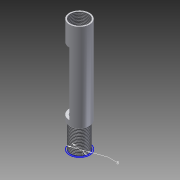
# Autodesk Inventor part: PEEKAufsatz1
Saved by Autodesk Inventor 2012 (Build 160160000, 160)
## iProperties
Created: 2014-06-23
Part Number: PEEKAufsatz1
Material: Polyaryletherketon-Kunststoff
Document SubType Name: Modeling
Designer: kathrin.ganzhorn
Density: 1.32 g/cm^3
Mass: 0.946631 g
Surface Area: 20.3493 cm^2
Volume: 0.717145 cm^3
Author: kathrin.ganzhorn
Autodesk Inventor part; units mm, degrees
ref_plane "YZ Plane" through (0, 0, 0) normal (1, 0, 0) x (0, 1, 0)
ref_plane "XZ Plane" through (0, 0, 0) normal (0, 1, 0) x (-1, 0, 0)
ref_plane "XY Plane" through (0, 0, 0) normal (0, 0, 1) x (1, 0, 0)
sketch "Skizze1" plane through (0, 0, 0) normal (0, 0, 1) x (1, 0, 0)
  circle A0 centre (0, 0) radius 4
  circle A1 centre (0, 0) radius 3.5
  dimension "d0" = 8
  dimension "d23" = 7
  constraints: 2 centre point, 2 coincident
  measures "d0" diameter of A0
  measures "d23" diameter of A1
extrude "Extrusion1" add sketch "Skizze1" along normal blind 45 contours A0 | A1
hole "Bohrung1" at (0, 0, 0) direction (0, 0, 1) diameter 6 end through all
extrude "Extrusion5" cut sketch "Skizze1" along normal blind 10
thread "Gewinde3" size "M7x0.5" class "6g" standard "ANSI Metric M Profile" full length
sketch "Skizze5" plane through (0, 0, 45) normal (0, 0, 1) x (1, 0, 0)
  circle A0 centre (0, 0) radius 4 projected
hole "Bohrung2" at (0, 0, 45) direction (0, 0, -1) diameter 7 depth 12 tip angle 118
thread "Gewinde4" size "M7x0.5" class "6H" standard "ANSI Metric M Profile" full length
sketch "Skizze6" plane through (0, 0, 0) normal (1, 0, 0) x (0, 1, 0)
  line L0 (5.1203, 12) -> (-6.2581, 12)
  line L1 (-6.2581, 12) -> (-6.2581, 37)
  line L2 (-6.2581, 37) -> (5.1203, 37)
  line L3 (5.1203, 37) -> (5.1203, 12)
  point P0 (0, 0)
  dimension "d37" = 25
  constraints: 8 end point, 2 parallel, 1 horizontal, 1 perpendicular
  measures "d37" distance of L0.end L1.end
extrude "Extrusion6" cut sketch "Skizze6" against normal blind 10
